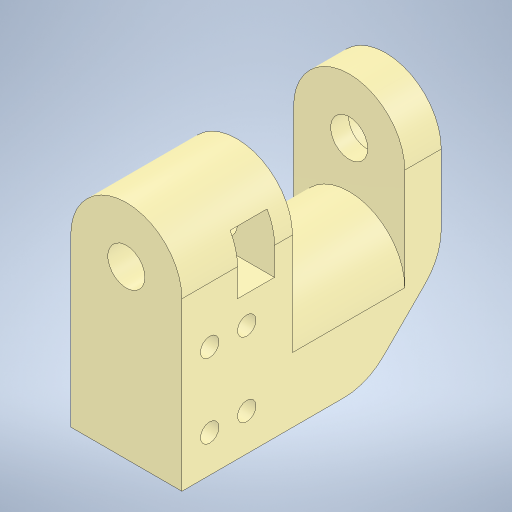
# Autodesk Inventor part: Side Mounts
Saved by Autodesk Inventor 2023.2 (Build 272271000, 271)
## iProperties
Created: 2024-04-13
Part Number: Side Mounts
Material: Nylon 6/6
Document SubType Name: Modeling
Designer: Nathan Cai
Mass: 24.1567 g
Surface Area: 64.6654 cm^2
Volume: 21.3776 cm^3
Density: 1.13 g/cm^3
Appearance: Nylon 6
Author: Nathan Cai
Autodesk Inventor part; units mm, degrees
ref_plane "YZ Plane" through (0, 0, 0) normal (1, 0, 0) x (0, 1, 0)
ref_plane "XZ Plane" through (0, 0, 0) normal (0, 1, 0) x (-1, 0, 0)
ref_plane "XY Plane" through (0, 0, 0) normal (0, 0, 1) x (1, 0, 0)
sketch "Sketch1" plane through (0, 0, 0) normal (1, 0, 0) x (0, 1, 0)
  line L0 (19.05, 22.225) -> (-19.05, 22.225)
  line L1 (-19.05, 22.225) -> (-19.05, -22.225)
  line L2 (-19.05, -22.225) -> (19.05, -22.225)
  line L3 (19.05, -22.225) -> (19.05, 22.225)
  line L4 (19.05, 22.225) -> (-19.05, -22.225) construction
  line L5 (-19.05, 22.225) -> (19.05, -22.225) construction
  line L6 (19.05, -15.875) -> (1.5875, -15.875)
  line L7 (1.5875, -15.875) -> (1.5875, 3.175)
  line L8 (1.5875, 3.175) -> (19.05, 3.175)
  line L9 (19.05, 3.175) -> (19.05, -15.875)
  line L10 (-19.05, 17.4625) -> (19.05, 17.4625) construction
  point P0 (0, 0)
  point P1 (-12.7, 17.4625)
  point P2 (0, 17.4625)
  point P3 (-12.7, 11.1125)
  point P4 (0, 11.1125)
  dimension "d0" = 38.1
  dimension "d1" = 44.45
  dimension "d2" = 17.4625
  dimension "d3" = 19.05
  dimension "d4" = 6.35
  dimension "d31" = 4.7625
  dimension "d32" = 6.35
  dimension "d35" = 12.7
  dimension "d38" = 6.35
  constraints: 22 end point, 4 parallel, 4 point on line, 3 horizontal, 3 perpendicular, 2 midpoint, 1 vertical, 3 other
  measures "d0" distance of L2.end L1.end
  measures "d1" distance of L1.end L0.end
  measures "d2" distance of L7.end L8.end
  measures "d3" distance of L6.end L7.end
  measures "d4" distance between parallel lines of L2 L6
  measures "d31" distance between parallel lines of L0 L10
  measures "d32" distance from line of L1 point (-12.7, 17.462)
  measures "d35" distance of point (-12.7, 17.462) point (0, 17.463)
  measures "d38" distance of point (-12.7, 17.462) point (-12.7, 11.113)
extrude "Extrusion1" add sketch "Sketch1" against normal blind 19.05 contours L3 L8 L7 L6 L2 L1 L0
sketch "Sketch2" plane through (0, -19.05, -22.225) normal (0, 0, -1) x (-1, 0, 0)
  line L0 (0, 38.1) -> (19.05, 38.1) projected
  line L1 (0, 0) -> (0, 38.1) projected
  point P0 (0, 19.05)
  point P1 (9.525, 28.575)
  dimension "d7" = 9.525
  dimension "d8" = 9.525
  measures "d7" distance from line of L0 point (9.525, 28.575)
  measures "d8" distance from line of L1 point (9.525, 28.575)
hole "Hole1" at (-9.525, 9.525, -22.225) direction (0, 0, 1) diameter 6.35 end through all counterbore diameter 9.525 counterbore depth 3.175
sketch "Sketch3" plane through (-19.05, 0, 0) normal (-1, 0, 0) x (0, 0, 1)
  line L0 (3.175, 6.35) -> (3.175, 12.7) projected
  line L1 (22.225, 12.7) -> (22.225, 6.35) projected
  line L2 (3.175, 6.35) -> (3.175, 12.7) projected
  line L3 (3.175, 19.05) -> (3.175, 1.5875) projected
  line L4 (3.175, 9.525) -> (22.225, 9.525) construction
  line L5 (22.225, -19.05) -> (22.225, 19.05) projected
  line L6 (22.225, 19.05) -> (3.175, 19.05) projected
  line L7 (12.7, 14.2875) -> (6.35, 14.2875)
  line L8 (6.35, 14.2875) -> (6.35, 4.7625)
  line L9 (6.35, 4.7625) -> (12.7, 4.7625)
  line L10 (12.7, 4.7625) -> (12.7, 14.2875)
  line L11 (12.7, 14.2875) -> (6.35, 4.7625) construction
  line L12 (6.35, 14.2875) -> (12.7, 4.7625) construction
  point P0 (0, 0)
  point P1 (9.525, 9.525)
  dimension "d16" = 9.525
  dimension "d17" = 6.35
  dimension "d18" = 9.525
  dimension "d19" = 3.175
  constraints: 14 end point, 3 point on line, 2 midpoint, 2 parallel, 2 perpendicular, 1 horizontal
  measures "d16" distance between parallel lines of L6 L4
  measures "d17" distance of L9.end L8.end
  measures "d18" distance of L8.end L7.end
  measures "d19" distance between parallel lines of L3 L8
extrude "Extrusion2" cut sketch "Sketch3" against normal through all
fillet "Fillet1" radius 9.525 6 edges at (0, 19.05, 12.7) (0, 19.05, -19.05) (-19.05, 19.05, -19.05) (-19.05, 19.05, 12.7) (-19.05, 1.5875, -6.35) (0, 1.5875, -6.35)
chamfer "Chamfer1" distance 12.7 angle 45 1 edges at (-9.525, -19.05, -22.225)
fillet "Fillet2" radius 9.525 2 edges at (-9.525, -6.35, -22.225) (-9.525, -19.05, -9.525)
thicken "Thicken1" operation add thickness 0.1 both sides no extend neighbours yes toward (0, 0, 1) faces at (-3.6754, 5.7159, 3.175)
thicken "Thicken2" operation add thickness 0.1 both sides no extend neighbours yes toward (0, 0, -1) faces at (-3.6754, 5.7159, -15.875)
hole "Hole2" at (0, -12.7, 17.4625) at (0, 0, 17.4625) at (0, -12.7, 11.1125) at (0, 0, 11.1125) direction (-1, 0, 0) diameter 3.175 end through all
body "Solid1"
